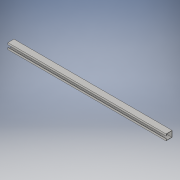
# Autodesk Inventor part: rail
Saved by Autodesk Inventor 2016 (Build 200138000, 138)
## iProperties
Created: 2017-08-29
Part Number: rail
Material: Generic
Document SubType Name: Modeling
Designer: m207653
Density: 1 g/cm^3
Appearance: Default
Author: m207653
Autodesk Inventor part; units mm, degrees
ref_plane "YZ Plane" through (0, 0, 0) normal (1, 0, 0) x (0, 1, 0)
ref_plane "XZ Plane" through (0, 0, 0) normal (0, 1, 0) x (-1, 0, 0)
ref_plane "XY Plane" through (0, 0, 0) normal (0, 0, 1) x (1, 0, 0)
sketch "Sketch1" plane through (0, 0, 0) normal (1, 0, 0) x (0, 1, 0)
  line L0 (0, 0) -> (50, 0)
  line L1 (50, 0) -> (50, 50)
  line L2 (50, 50) -> (0, 50)
  line L3 (0, 50) -> (0, 0)
  line L4 (0, 25) -> (0, 35)
  line L5 (0, 35) -> (4.6846, 35)
  line L6 (4.6846, 35) -> (4.6846, 15)
  line L7 (4.6846, 15) -> (0, 15)
  line L8 (0, 15) -> (0, 35)
  dimension "d0" = 50
  dimension "d1" = 50
  dimension "d2" = 10
  dimension "d3" = 20
  constraints: 18 end point, 4 perpendicular, 2 parallel, 2 point on line, 1 collinear, 1 horizontal, 1 midpoint
  measures "d0" distance of L2.end L1.end
  measures "d1" distance of L1.end L0.end
  measures "d2" distance of L4.start L4.end
  measures "d3" distance of L5.end L6.end
extrude "Extrusion1" add sketch "Sketch1" against normal blind 1300 contours L3 L7 L6 L5 L2 L1 L0
sketch "Sketch2" plane through (0, 0, 0) normal (1, 0, 0) x (0, 0, -1)
  line L0 (-47, 3) -> (-3, 3)
  line L1 (-3, 3) -> (-3, 47)
  line L2 (-3, 47) -> (-47, 47)
  line L3 (-47, 47) -> (-47, 3)
  line L4 (-50, 0) -> (-50, 50) projected
  line L5 (0, 50) -> (-50, 50) projected
  line L6 (0, 50) -> (0, 0) projected
  line L7 (-35, 0) -> (-50, 0) projected
  dimension "d6" = 3
  dimension "d7" = 3
  dimension "d8" = 3
  dimension "d9" = 3
  constraints: 8 end point, 2 parallel, 1 horizontal, 1 perpendicular
  measures "d6" distance between parallel lines of L4 L3
  measures "d7" distance between parallel lines of L5 L2
  measures "d8" distance between parallel lines of L6 L1
  measures "d9" distance between parallel lines of L7 L0
extrude "Extrusion2" cut sketch "Sketch2" against normal blind 1300
body "Solid1"
